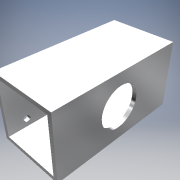
# Autodesk Inventor part: Arm 4 inch
Saved by Autodesk Inventor 2019 (Build 230136000, 136)
## iProperties
Created: 2018-09-22
Part Number: Arm 4 inch
Material: Aluminum 6061
Document SubType Name: Modeling
Designer: Adhik
Density: 2.7 g/cm^3
Appearance: Aluminum - Flat
Mass: 152.345 g
Surface Area: 373.857 cm^2
Volume: 56.424 cm^3
Author: Adhik
Autodesk Inventor part; units mm, degrees
ref_plane "YZ Plane" through (0, 0, 0) normal (1, 0, 0) x (0, 1, 0)
ref_plane "XZ Plane" through (0, 0, 0) normal (0, 1, 0) x (-1, 0, 0)
ref_plane "XY Plane" through (0, 0, 0) normal (0, 0, 1) x (1, 0, 0)
sketch "Sketch1" plane through (0, 0, 0) normal (0, 0, 1) x (1, 0, 0)
  line L0 (-35.56, 0) -> (35.56, 0) construction
  line L1 (0, -35.56) -> (0, 35.56) construction
  line L2 (-25.4, 25.4) -> (25.4, 25.4)
  line L3 (25.4, 25.4) -> (25.4, -25.4)
  line L4 (25.4, -25.4) -> (-25.4, -25.4)
  line L5 (-25.4, -25.4) -> (-25.4, 25.4)
  line L6 (-22.225, 22.225) -> (22.225, 22.225)
  line L7 (22.225, 22.225) -> (22.225, -22.225)
  line L8 (22.225, -22.225) -> (-22.225, -22.225)
  line L9 (-22.225, -22.225) -> (-22.225, 22.225)
  point P0 (0, 0)
  point P1 (-25.4, 0)
  point P2 (0, 25.4)
  point P3 (-22.225, 0)
  point P4 (0, 22.225)
  dimension "d0" = 50.8
  dimension "d1" = 3.175
  dimension "d11" = 50.8
  dimension "d12" = 3.175
  constraints: 16 end point, 4 midpoint, 4 parallel, 4 point on line, 2 horizontal, 2 perpendicular
  measures "d0" distance of L4.end L2.start
  measures "d1" distance between parallel lines of L2 L6
  measures "d11" distance of L2.start L2.end
  measures "d12" distance between parallel lines of L5 L9
extrude "Extrusion1" add sketch "Sketch1" along normal mid plane 101.6
sketch "Sketch6" plane through (25.4, -25.4, 50.8) normal (1, 0, 0) x (0, 0, -1)
  circle A0 centre (50.8, 25.4) radius 14.2875
  dimension "d23" = 28.575
  constraints: 1 centre point, 1 coincident
  measures "d23" diameter of A0
extrude "Extrusion7" cut sketch "Sketch6" against normal through all
sketch "Sketch7" plane through (-22.225, -22.225, -50.8) normal (1, 0, 0) x (0, 0, -1)
  circle A0 centre (-14.8971, 6.35) radius 2.667 projected
  circle A1 centre (-86.7029, 6.35) radius 2.667 projected
  circle A2 centre (-14.8971, 38.1) radius 2.667 projected
  circle A3 centre (-86.7029, 38.1) radius 2.667 projected
  point P0 (-50.8, 22.225)
extrude "Extrusion8" cut sketch "Sketch7" against normal up to next
sketch "Sketch8" plane through (25.4, -25.4, 50.8) normal (1, 0, 0) x (0, 0, -1)
  circle A0 centre (50.8, 25.4) radius 15.875 construction
  line L0 (121.92, 25.4) -> (-20.32, 25.4) construction
  circle A1 centre (69.85, 25.4) radius 3.175 construction
  line L1 (50.8, 9.525) -> (50.8, 41.275) construction
  circle A2 centre (69.85, 25.4) radius 5.5499 construction
  circle A3 centre (69.85, 25.4) radius 2.667
  circle A4 centre (31.75, 25.4) radius 2.667
  point P0 (50.8, 25.4)
  dimension "d28" = 6.35
  dimension "d29" = 11.0998
  dimension "d30" = 5.334
  constraints: 4 centre point, 2 coincident, 2 end point, 2 point on circle, 1 midpoint, 1 point on line, 1 symmetric about line, 1 tangent, 1 vertical, 1 other
  measures "d28" diameter of A1
  measures "d29" diameter of A2
  measures "d30" diameter of A3
extrude "Extrusion9" cut sketch "Sketch8" against normal through all
equation "\"d12\" = d1"
body "Solid1"
